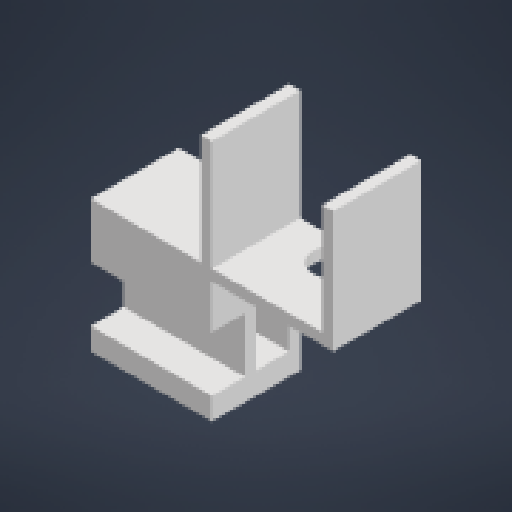
# Autodesk Inventor part: Part56
Saved by Autodesk Inventor 2027.1 (Build 311270010, 270A)
## iProperties
Created: 2026-09-29
Part Number: Part56
Material: Generic
Document SubType Name: Modeling
Designer: daniel
Density: 1 g/cm^3
Appearance: Default
Author: daniel
Autodesk Inventor part; units mm, degrees
ref_plane "YZ Plane" through (0, 0, 0) normal (1, 0, 0) x (0, 1, 0)
ref_plane "XZ Plane" through (0, 0, 0) normal (0, 1, 0) x (-1, 0, 0)
ref_plane "XY Plane" through (0, 0, 0) normal (0, 0, 1) x (1, 0, 0)
sketch "Sketch1" plane through (0, 0, 0) normal (0, 0, 1) x (1, 0, 0)
  line L0 (-25, 25) -> (25, 25)
  line L1 (25, 25) -> (25, -30)
  line L2 (30, -25) -> (-30, -25)
  line L3 (-25, -30) -> (-25, 80)
  line L4 (-25, 25) -> (25, -25) construction
  line L5 (25, 25) -> (-25, -25) construction
  line L6 (25, 25) -> (-51, 25)
  line L7 (25, 80) -> (25, 25)
  line L8 (-51, 25) -> (-75, 25)
  line L9 (-75, 25) -> (-75, -25)
  line L10 (-75, -25) -> (-30, -25)
  line L11 (30, 30) -> (-30, 30)
  line L12 (-30, 30) -> (-30, -30)
  line L13 (-30, -30) -> (30, -30)
  line L14 (30, -30) -> (30, 30)
  line L15 (30, 25) -> (30, 80)
  line L16 (-30, 80) -> (-30, 25)
  line L17 (-80, -30) -> (-80, 30)
  line L18 (-80, 30) -> (-30, 30)
  line L19 (-30, -30) -> (-80, -30)
  line L20 (-30, 80) -> (30, 80)
  line L21 (24.924, 24.924) -> (30, 25)
  point P0 (0, 0)
  point P1 (25, 30)
  point P2 (-30, 25)
  point P3 (-25, 30)
  point P4 (25, 24.9251)
  dimension "d4" = 5
  dimension "d7" = 50
  dimension "d8" = 0
  dimension "d9" = 5
  dimension "d12" = 55
  dimension "d13" = 60
  dimension "d14" = 105
  dimension "d15" = 50
  dimension "d18" = 110
  dimension "d19" = 3.5355
  dimension "d20" = 38.8909
  dimension "d21" = 81
  constraints: 44 end point, 11 point on line, 7 parallel, 5 perpendicular, 4 horizontal, 3 midpoint
  measures "d4" distance between parallel lines of L0 L11
  measures "d7" distance between parallel lines of L17 L12
  measures "d8" distance between parallel lines of L15 L14
  measures "d9" distance between parallel lines of L15 L1
  measures "d12" distance between parallel lines of L15 L3
  measures "d13" distance between parallel lines of L15 L12
  measures "d14" distance between parallel lines of L15 L9
  measures "d15" distance between parallel lines of L20 L11
  measures "d18" distance between parallel lines of L20 L13
  measures "d19" distance from line of L15.start L5
  measures "d20" distance from line of L16.end L5
  measures "d21" distance from line of L6.end L15
extrude "Extrusion1" add sketch "Sketch1" along normal blind 40 contours L3 L11 L7 L0 | L6 L12 L11 L3 | L3 L2 L12 L6 | L7 L11 L14 L21 L1 | L3 L13 L12 L2 | L11 L16 L20 L3 | L12 L10 L9 L8 L6 | L6 L8 L9 L10 L12 L19 L17 L18 | L7 L20 L15 L11
sketch "Sketch2" plane through (-25, 25, 0) normal (0, -1, 0) x (1, 0, 0)
  circle A0 centre (25, 13) radius 9
  line L0 (0, 0) -> (50, 0) projected
  point P0 (25, 0)
  dimension "d24" = 18
  dimension "d25" = 13
  constraints: 1 centre point
  measures "d24" diameter of A0
  measures "d25" distance from line of L0 A0.centre
extrude "Extrusion2" cut sketch "Sketch2" against normal blind 40
sketch "Sketch3" plane through (-25, -30, 0) normal (1, 0, 0) x (0, 0, -1)
  line L0 (0, 0) -> (-40, 0) projected
  line L1 (0, 55) -> (-40, 55) projected
  line L2 (0, 0) -> (-5, 0)
  line L3 (-5, 0) -> (-5, 55)
  line L4 (-5, 55) -> (0, 55)
  line L5 (0, 55) -> (0, 0)
  line L6 (-5, 0) -> (-20, 0)
  line L7 (-20, 0) -> (-20, 55)
  line L8 (-20, 55) -> (-5, 55)
  line L9 (-5, 55) -> (-5, 0)
  line L10 (-20, 0) -> (-25, 0)
  line L11 (-25, 0) -> (-25, 55)
  line L12 (-25, 55) -> (-20, 55)
  line L13 (-20, 55) -> (-20, 0)
  line L14 (-25, 0) -> (-40, 0)
  line L15 (-40, 0) -> (-40, 55)
  line L16 (-40, 55) -> (-25, 55)
  line L17 (-25, 55) -> (-25, 0)
  line L18 (-40, 0) -> (0, 0)
  line L19 (0, 0) -> (0, 10)
  line L20 (0, 10) -> (-40, 10)
  line L21 (-40, 10) -> (-40, 0)
  line L22 (-40, 55) -> (-20, 55)
  line L23 (-20, 55) -> (-20, 37.9712)
  line L24 (-20, 37.9712) -> (-40, 37.9712)
  line L25 (-40, 37.9712) -> (-40, 55)
  line L26 (-40, 55) -> (-5, 55)
  line L27 (-5, 55) -> (-5, 35)
  line L28 (-5, 35) -> (-40, 35)
  line L29 (-40, 35) -> (-40, 55)
  point P0 (0, 30)
  point P1 (-20, 10)
  point P2 (-5, 10)
  point P3 (-25, 10)
  point P4 (-20, 35)
  point P5 (-25, 35)
  dimension "d28" = 5
  dimension "d29" = 15
  dimension "d30" = 5
  dimension "d33" = 10
  dimension "d34" = 20
  dimension "d35" = 20
  constraints: 56 end point, 14 parallel, 7 horizontal, 7 perpendicular, 4 point on line, 1 midpoint
  measures "d28" distance of L3.end L4.end
  measures "d29" distance of L7.end L8.end
  measures "d30" distance of L11.end L12.end
  measures "d33" distance of L19.end L18.end
  measures "d34" distance of L23.end L24.end
  measures "d35" distance of L26.end L27.end
extrude "Extrusion3" cut sketch "Sketch3" against normal through all contours L20 L7 L28 L3 | L20 L15 L28 L11
body "Solid1"
